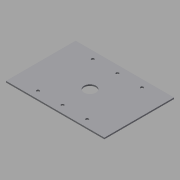
# Autodesk Inventor part: Mounting Plate
Saved by Autodesk Inventor 2013 (Build 170138000, 138)
## iProperties
Created: 2013-02-08
Part Number: Mounting Plate
Material: Generic
Document SubType Name: Modeling
Designer: Naphat
Density: 1 g/cm^3
Author: Naphat
Autodesk Inventor part; units mm, degrees
ref_plane "YZ Plane" through (0, 0, 0) normal (1, 0, 0) x (0, 1, 0)
ref_plane "XZ Plane" through (0, 0, 0) normal (0, 1, 0) x (-1, 0, 0)
ref_plane "XY Plane" through (0, 0, 0) normal (0, 0, 1) x (1, 0, 0)
sketch "Sketch1" plane through (0, 0, 0) normal (0, 1, 0) x (-1, 0, 0)
  line L0 (0, 0) -> (213.36, 0)
  line L1 (213.36, 0) -> (213.36, 151.003)
  line L2 (213.36, 151.003) -> (0, 151.003)
  line L3 (0, 151.003) -> (0, 0)
  dimension "d0" = 213.36
  dimension "d1" = 151.003
  constraints: 8 end point, 2 perpendicular, 1 horizontal, 1 parallel
  measures "d0" distance of L0.start L0.end
  measures "d1" distance of L0.end L1.end
extrude "Extrusion1" add sketch "Sketch1" along normal blind 3
sketch "Sketch2" plane through (0, 3, 0) normal (0, 1, 0) x (1, 0, 0)
  line L0 (0, 0) -> (-213.36, 0) projected
  line L1 (-213.36, 0) -> (-213.36, -151.003) projected
  line L2 (-213.36, -151.003) -> (0, -151.003) projected
  line L3 (0, -151.003) -> (0, 0) projected
  line L4 (-213.36, 0) -> (-213.36, -75.5015) construction
  line L5 (-213.36, -75.5015) -> (0, -75.5015) construction
  line L6 (-213.36, 0) -> (-106.68, 0) construction
  line L7 (-106.68, 0) -> (-106.68, -151.003) construction
  circle A0 centre (-106.68, -75.5015) radius 13.0048
  dimension "d4" = 75.5015
  dimension "d5" = 151.003
  dimension "d6" = 213.36
  dimension "d7" = 106.68
  dimension "d8" = 26.0096
  constraints: 8 end point, 5 midpoint, 1 centre point
  measures "d4" distance of L0.end L4.end
  measures "d5" distance of L0.end L1.end
  measures "d6" distance of L0.start L0.end
  measures "d7" distance of L0.end L6.end
  measures "d8" diameter of A0
hole "Hole1" at (-106.68, 3, 75.5015) direction (0, -1, 0) diameter 26.0096 depth 25.4 tip angle 118
sketch "Sketch3" plane through (0, 3, 0) normal (0, 1, 0) x (1, 0, 0)
  line L0 (0, 0) -> (-213.36, 0) projected
  line L1 (-213.36, 0) -> (-213.36, -151.003) projected
  line L2 (-213.36, -151.003) -> (0, -151.003) projected
  line L3 (0, -151.003) -> (0, 0) projected
  line L4 (-213.36, 0) -> (-213.36, -16) construction
  line L5 (-213.36, -16) -> (0, -16) construction
  line L6 (-213.36, -16) -> (-160.02, -16) construction
  line L7 (-160.02, -16) -> (-106.68, -16) construction
  line L8 (-106.68, -16) -> (-53.34, -16) construction
  line L9 (-53.34, -16) -> (0, -16) construction
  line L10 (-213.36, -151.003) -> (-213.36, -135.003) construction
  line L11 (-213.36, -135.003) -> (0, -135.003) construction
  line L12 (-160.02, 0) -> (-160.02, -151.003) construction
  line L13 (-106.68, 0) -> (-106.68, -151.003) construction
  line L14 (-53.34, 0) -> (-53.34, -151.003) construction
  circle A0 centre (-160.02, -135.003) radius 3.175
  circle A1 centre (-106.68, -135.003) radius 3.175
  circle A2 centre (-53.34, -135.003) radius 3.175
  circle A3 centre (-53.34, -16) radius 3.175
  circle A4 centre (-106.68, -16) radius 3.175
  circle A5 centre (-160.02, -16) radius 3.175
  dimension "d16" = 16
  dimension "d17" = 213.36
  dimension "d18" = 53.34
  dimension "d19" = 53.34
  dimension "d20" = 53.34
  dimension "d21" = 53.34
  dimension "d22" = 16
  dimension "d23" = 6.35
  dimension "d24" = 6.35
  dimension "d25" = 6.35
  dimension "d26" = 6.35
  dimension "d27" = 6.35
  dimension "d28" = 6.35
  constraints: 22 end point, 15 point on line, 6 centre point, 5 perpendicular, 4 midpoint, 3 coincident
  measures "d16" distance of L0.end L4.end
  measures "d17" distance of L4.end L5.end
  measures "d18" distance of L4.end L6.end
  measures "d19" distance of L6.end L7.end
  measures "d20" distance of L7.end L8.end
  measures "d21" distance of L8.end L5.end
  measures "d22" distance of L1.end L10.end
  measures "d23" diameter of A5
  measures "d24" diameter of A4
  measures "d25" diameter of A3
  measures "d26" diameter of A2
  measures "d27" diameter of A1
  measures "d28" diameter of A0
hole "Hole2" at (-53.34, 3, 135.003) at (-106.68, 3, 135.003) at (-160.02, 3, 135.003) at (-160.02, 3, 16) at (-106.68, 3, 16) at (-53.34, 3, 16) direction (0, -1, 0) diameter 6.35 depth 25.4 tip angle 118
equation "\"d4\" = 0.5 * d5"
equation "\"d7\" = 0.5 * d6"
equation "\"d19\" = d18"
equation "\"d20\" = d18"
equation "\"d24\" = d23"
equation "\"d25\" = d24"
equation "\"d26\" = d25"
equation "\"d27\" = d25"
equation "\"d28\" = d27"
body "Solid1"
